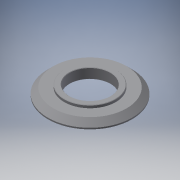
# Autodesk Inventor part: KM-20140709-07-Kashiyama 機械油封墊片(T=7.5)
Saved by Autodesk Inventor 2018 (Build 220112000, 112)
## iProperties
Created: 2014-07-10
Part Number: KM-20140709-07-Kashiyama 機械油封墊片(T=7.5)
Material: 一般
Document SubType Name: Modeling
Designer: ERIC
Density: 1 g/cm^3
Appearance: 預設
Author: ERIC
Autodesk Inventor part; units mm, degrees
ref_plane "YZ Plane" through (0, 0, 0) normal (1, 0, 0) x (0, 1, 0)
ref_plane "XZ Plane" through (0, 0, 0) normal (0, 1, 0) x (-1, 0, 0)
ref_plane "XY Plane" through (0, 0, 0) normal (0, 0, 1) x (1, 0, 0)
sketch "草圖1" plane through (0, 0, 0) normal (0, 0, 1) x (1, 0, 0)
  circle A0 centre (0, 0) radius 31
  dimension "d0" = 62
  constraints: 1 centre point, 1 coincident
  measures "d0" diameter of A0
extrude "擠出1" add sketch "草圖1" along normal blind 1
sketch "草圖2" plane through (0, 0, 1) normal (0, 0, 1) x (1, 0, 0)
  circle A0 centre (0, 0) radius 31 projected
  circle A1 centre (0, 0) radius 27
  dimension "d3" = 54
  constraints: 1 centre point, 1 coincident
  measures "d3" diameter of A1
extrude "擠出2" add sketch "草圖2" along normal blind 4 contours A1
sketch "草圖3" plane through (0, 0, 5) normal (0, 0, 1) x (1, 0, 0)
  circle A0 centre (0, 0) radius 27 projected
  circle A1 centre (0, 0) radius 19
  dimension "d6" = 38
  constraints: 1 centre point, 1 coincident
  measures "d6" diameter of A1
extrude "擠出3" add sketch "草圖3" along normal blind 2 contours A1
sketch "草圖4" plane through (0, 0, 0) normal (0, 0, -1) x (-1, 0, 0)
  circle A0 centre (0, 0) radius 31 projected
  circle A1 centre (0, 0) radius 20
  dimension "d9" = 40
  constraints: 1 centre point, 1 coincident
  measures "d9" diameter of A1
extrude "擠出4" add sketch "草圖4" along normal blind 0.5 contours A1
sketch "草圖5" plane through (0, 0, 7) normal (0, 0, 1) x (1, 0, 0)
  circle A0 centre (0, 0) radius 19 projected
  circle A1 centre (0, 0) radius 15
  dimension "d12" = 30
  constraints: 1 centre point, 1 coincident
  measures "d12" diameter of A1
extrude "擠出5" cut sketch "草圖5" against normal through all contours A1
chamfer "倒角1" distance 4 angle 45 1 edges at (-27, 0, 1)
chamfer "倒角2" distance 0.3 angle 45 3 edges at (-15, 0, 7) (-15, 0, -0.5) (-19, 0, 7)
